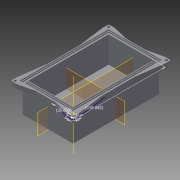
# Autodesk Inventor part: sensor3_2
Saved by Autodesk Inventor 2015 SP2 (Build 190223200, 223)
## iProperties
Created: 2016-02-03
Part Number: sensor3_2
Material: Generic
Document SubType Name: Modeling
Designer: mca20
Density: 1 g/cm^3
Appearance: Default
Author: mca20
Autodesk Inventor part; units mm, degrees
ref_plane "YZ Plane" through (0, 0, 0) normal (1, 0, 0) x (0, 1, 0)
ref_plane "XZ Plane" through (0, 0, 0) normal (0, 1, 0) x (-1, 0, 0)
ref_plane "XY Plane" through (0, 0, 0) normal (0, 0, 1) x (1, 0, 0)
sketch "Sketch1" plane through (0, 0, 0) normal (0, 1, 0) x (-1, 0, 0)
  line L0 (0, 0) -> (69.34, 0)
  line L1 (69.34, 0) -> (69.34, -118.083)
  line L2 (69.34, -118.083) -> (0, -118.083)
  line L3 (0, -118.083) -> (0, 0)
  dimension "d0" = 69.34
  dimension "d1" = 118.083
  constraints: 8 end point, 2 parallel, 1 horizontal, 1 perpendicular
  measures "d0" distance of L1.end L2.end
  measures "d1" distance of L0.end L1.end
extrude "Extrusion1" add sketch "Sketch1" along normal blind 1
sketch "Sketch2" plane through (0, 1, 0) normal (0, 1, 0) x (1, 0, 0)
  line L0 (0, 0) -> (0, 118.083) projected
  line L1 (-69.34, 0) -> (0, 0) projected
  line L2 (0, 0) -> (0, 118.083) projected
  line L3 (0, 118.083) -> (-69.34, 118.083) projected
  line L4 (-69.34, 118.083) -> (-69.34, 0) projected
  line L5 (-68.34, 1) -> (-1, 1)
  line L6 (-1, 1) -> (-1, 117.083)
  line L7 (-1, 117.083) -> (-68.34, 117.083)
  line L8 (-68.34, 117.083) -> (-68.34, 1)
  dimension "d4" = 1
  constraints: 8 end point, 3 other
  measures "d4" distance between parallel lines of L4 L8
extrude "Extrusion2" add sketch "Sketch2" along normal blind 35
sketch "Sketch3" plane through (0, 36, 0) normal (0, 1, 0) x (1, 0, 0)
  line L0 (-68.34, 1) -> (-68.34, 117.083) projected
  line L1 (-68.34, 117.083) -> (-1, 117.083) projected
  line L2 (-1, 117.083) -> (-1, 1) projected
  line L3 (-1, 1) -> (-68.34, 1) projected
  line L4 (-69.34, 0) -> (0, 0) projected
  line L5 (0, 0) -> (0, 118.083) projected
  line L6 (0, 118.083) -> (-69.34, 118.083) projected
  line L7 (-69.34, 118.083) -> (-69.34, 0) projected
  line L8 (-67.34, 116.083) -> (-67.34, 2)
  line L9 (-67.34, 2) -> (-2, 2)
  line L10 (-2, 2) -> (-2, 116.083)
  line L11 (-2, 116.083) -> (-67.34, 116.083)
  line L12 (-66.34, 3) -> (-66.34, 115.083)
  line L13 (-66.34, 115.083) -> (-3, 115.083)
  line L14 (-3, 115.083) -> (-3, 3)
  line L15 (-3, 3) -> (-66.34, 3)
  line L16 (-70.34, -1) -> (1, -1)
  line L17 (1, -1) -> (1, 119.083)
  line L18 (1, 119.083) -> (-70.34, 119.083)
  line L19 (-70.34, 119.083) -> (-70.34, -1)
  line L20 (-71.34, -2) -> (2, -2)
  line L21 (2, -2) -> (2, 120.083)
  line L22 (2, 120.083) -> (-71.34, 120.083)
  line L23 (-71.34, 120.083) -> (-71.34, -2)
  dimension "d7" = 1
  dimension "d8" = 1
  dimension "d9" = 1
  dimension "d10" = 1
  constraints: 32 end point, 12 other
  measures "d7" distance between parallel lines of L0 L8
  measures "d8" distance between parallel lines of L8 L12
  measures "d9" distance between parallel lines of L7 L19
  measures "d10" distance between parallel lines of L19 L23
extrude "Extrusion3" add sketch "Sketch3" along normal blind 1 contours L0 L1 L2 L3 | L7 L6 L5 L4 | L11 L10 L9 L8 | L19 L18 L17 L16 | L23 L22 L21 L20
sketch "Sketch4" plane through (0, 37, 0) normal (0, 1, 0) x (1, 0, 0)
  line L0 (-71.34, 120.083) -> (-71.34, -2) projected
  line L1 (-66.34, 3) -> (-66.34, 115.083) projected
  line L2 (-66.34, 115.083) -> (-3, 115.083) projected
  line L3 (-3, 115.083) -> (-3, 3) projected
  line L4 (-3, 3) -> (-66.34, 3) projected
  line L5 (-66.34, 3) -> (-66.34, 115.083) projected
  line L6 (-71.34, -2) -> (2, -2) projected
  line L7 (2, -2) -> (2, 120.083) projected
  line L8 (2, 120.083) -> (-71.34, 120.083) projected
  line L9 (-71.34, 120.083) -> (-71.34, -2) projected
  line L10 (-1, 1) -> (-68.34, 1) projected
  line L11 (-69.34, 0) -> (0, 0) projected
  line L12 (-69.34, 118.083) -> (-69.34, 0) projected
  line L13 (-68.34, 1) -> (-68.34, 117.083) projected
  line L14 (-1, 117.083) -> (-1, 1) projected
  line L15 (0, 0) -> (0, 118.083) projected
  line L16 (-68.34, 117.083) -> (-1, 117.083) projected
  line L17 (0, 118.083) -> (-69.34, 118.083) projected
  line L18 (-70.34, 119.083) -> (-70.34, -1)
  line L19 (-70.34, -1) -> (1, -1)
  line L20 (1, -1) -> (1, 119.083)
  line L21 (1, 119.083) -> (-70.34, 119.083)
  line L22 (-2, 116.083) -> (-67.34, 116.083)
  line L23 (-67.34, 116.083) -> (-67.34, 2)
  line L24 (-67.34, 2) -> (-2, 2)
  line L25 (-2, 2) -> (-2, 116.083)
  dimension "d13" = 1
  dimension "d14" = 1
  constraints: 16 end point, 6 other
  measures "d13" distance between parallel lines of L17 L21
  measures "d14" distance between parallel lines of L2 L22
extrude "Extrusion4" add sketch "Sketch4" along normal blind 1.5 contours L8 L7 L6 L0 | L25 L24 L23 L22
sketch "Sketch10" plane through (0, 37, 0) normal (0, 1, 0) x (1, 0, 0)
  line L0 (-71.34, -2) -> (2, -2) projected
  line L1 (-67.34, 2) -> (-2, 2) projected
  line L2 (-70.34, 119.083) -> (1, 119.083) projected
  line L3 (1, 119.083) -> (1, -1) projected
  line L4 (1, -1) -> (-70.34, -1) projected
  line L5 (-70.34, -1) -> (-70.34, 119.083) projected
  line L6 (-71.34, -2) -> (2, -2) projected
  line L7 (2, -2) -> (2, 120.083) projected
  line L8 (2, 120.083) -> (-71.34, 120.083) projected
  line L9 (-71.34, 120.083) -> (-71.34, -2) projected
  line L10 (-1, 1) -> (-68.34, 1) projected
  line L11 (-2, 116.083) -> (-2, 2) projected
  line L12 (-2, 2) -> (-67.34, 2) projected
  line L13 (-67.34, 2) -> (-67.34, 116.083) projected
  line L14 (-67.34, 116.083) -> (-2, 116.083) projected
  line L15 (1, 119.083) -> (-70.34, 119.083) projected
  line L16 (-70.34, 119.083) -> (-70.34, -1) projected
  line L17 (-70.34, -1) -> (1, -1) projected
  line L18 (1, -1) -> (1, 119.083) projected
  line L19 (-68.34, 1) -> (-68.34, 117.083) projected
  line L20 (-1, 117.083) -> (-1, 1) projected
  line L21 (1, 119.083) -> (1, -1) projected
  line L22 (0, 0) -> (0, 118.083) projected
  line L23 (-69.34, 0) -> (0, 0) projected
  line L24 (-69.34, 118.083) -> (-69.34, 0) projected
  line L25 (-2, 116.083) -> (-67.34, 116.083) projected
  line L26 (-68.34, 117.083) -> (-1, 117.083) projected
  line L27 (0, 118.083) -> (-69.34, 118.083) projected
  line L28 (-72.34, 121.083) -> (3, 121.083)
  line L29 (3, 121.083) -> (3, -3)
  line L30 (3, -3) -> (-72.34, -3)
  line L31 (-72.34, -3) -> (-72.34, 121.083)
  line L32 (-3, 115.083) -> (-3, 3) projected
  line L33 (-3, 3) -> (-66.34, 3) projected
  line L34 (-66.34, 3) -> (-66.34, 115.083) projected
  line L35 (-66.34, 115.083) -> (-3, 115.083) projected
  line L36 (-2, 116.083) -> (-67.34, 116.083) projected
  line L37 (-67.34, 116.083) -> (-67.34, 2) projected
  line L38 (-67.34, 2) -> (-2, 2) projected
  line L39 (-2, 2) -> (-2, 116.083) projected
  line L40 (-65.34, 114.083) -> (-65.34, 4)
  line L41 (-65.34, 4) -> (-4, 4)
  line L42 (-4, 4) -> (-4, 114.083)
  line L43 (-4, 114.083) -> (-65.34, 114.083)
  dimension "d50" = 1
  dimension "d51" = 1
  dimension "d69" = 61.34
  dimension "d70" = 110.083
  constraints: 16 end point, 6 other
  measures "d50" distance between parallel lines of L8 L28
  measures "d51" distance between parallel lines of L34 L40
  measures "d69" distance between parallel lines of L42 L40
  measures "d70" distance between parallel lines of L41 L43
extrude "Extrusion6" add sketch "Sketch10" along normal blind 3 and the other way blind 1 contours L28 L29 L30 L31 | L32 L33 L34 L35
sketch "Sketch5" plane through (0, 36, 0) normal (0, -1, 0) x (1, 0, 0)
  line L0 (0, 0) -> (8, 0)
  line L1 (8, 0) -> (8, 8)
  line L2 (8, 8) -> (0, 8)
  line L3 (0, 8) -> (0, 0)
  line L4 (8, 8) -> (2, 8)
  line L5 (2, 8) -> (2, 2)
  line L6 (2, 2) -> (8, 2)
  line L7 (8, 2) -> (8, 8)
  line L8 (0, 0) -> (0, -118.083) projected
  line L9 (0, -59.0415) -> (8, 0)
  line L10 (-69.34, 0) -> (0, 0) projected
  line L11 (-34.67, 0) -> (0, 8)
  circle A0 centre (5, 5) radius 1.5
  line L12 (7, 3) -> (3, 3)
  line L13 (3, 3) -> (3, 7)
  line L14 (3, 7) -> (7, 7)
  line L15 (7, 7) -> (7, 3)
  line L16 (-71.34, 2) -> (2, 2) projected
  line L17 (-26.0025, 2) -> (-26.0025, 0)
  line L18 (-26.0025, 2) -> (-16.75, 2) construction
  dimension "d17" = 8
  dimension "d18" = 8
  dimension "d21" = 6
  dimension "d29" = 118.083
  dimension "d31" = 3
  dimension "d32" = 1
  dimension "d47" = 26.0025
  constraints: 32 end point, 6 parallel, 4 perpendicular, 3 horizontal, 3 point on line, 2 midpoint, 1 centre point, 1 coincident, 3 other
  measures "d17" distance of L2.end L1.end
  measures "d18" distance of L1.end L0.end
  measures "d21" distance between parallel lines of L2 L6
  measures "d29" distance of L0.start L8.end
  measures "d31" diameter of A0
  measures "d32" distance between parallel lines of L6 L12
  measures "d47" distance between parallel lines of L3 L17
extrude "Extrusion5" add sketch "Sketch5" along normal blind 2 contours L3 L16 L6 L1 L0 | L10 L17 L16 L3 | L0 L9 L8 | L16 L11 L3 | L3 L2 L5 L16 | L10 L11 L17 | L6 L5 L2 L1 | A0 | L12 L13 L14 L15
sketch "Sketch6" plane through (0, 36, 0) normal (0, 1, 0) x (1, 0, 0)
  line L0 (8, -8) -> (0, -8) projected
  line L1 (8, -8) -> (0, -8) projected
  line L2 (8, 0) -> (8, -8) projected
  line L3 (8, -8) -> (2, -8)
  line L4 (2, -8) -> (2, -2)
  line L5 (2, -2) -> (8, -2)
  line L6 (8, -2) -> (8, -8)
  line L7 (0, -8) -> (-21.6687, -3) projected
  line L8 (3, 36.9009) -> (8, 0) projected
  line L9 (3, 36.9009) -> (3, -3) projected
  line L10 (3, -3) -> (-21.6687, -3) projected
  point P0 (0, 0)
  point P1 (5, -5)
  dimension "d33" = 3
  dimension "d34" = 6
  dimension "d35" = 3
  dimension "d36" = 3
  constraints: 8 end point, 2 parallel, 1 horizontal, 1 perpendicular
  measures "d33" distance from line of L5 point (5, -5)
  measures "d34" distance between parallel lines of L5 L0
  measures "d35" distance from line of L2 point (5, -5)
  measures "d36" distance from line of L0 point (5, -5)
hole "Hole1" at (5, 36, 5) direction (0, -1, 0) diameter 3 end through all
fillet "Fillet1" radius 2 1 edges at (8, 35, 8)
sketch "Sketch11" plane through (0, 36, 0) normal (0, 1, 0) x (1, 0, 0)
  line L0 (8, -8) -> (2, -8)
  line L1 (2, -8) -> (2, -2)
  line L2 (2, -2) -> (8, -2)
  line L3 (8, -2) -> (8, -8)
  line L4 (0, 0) -> (8, 0)
  line L5 (8, 0) -> (8, -8)
  line L6 (8, -8) -> (0, -8)
  line L7 (0, -8) -> (0, 0)
  line L8 (-21.6687, -3) -> (0, -8)
  line L9 (0, -8) -> (-21.6687, -3) projected
  line L10 (-21.6687, -3) -> (0, -3)
  line L11 (3, -3) -> (-21.6687, -3) projected
  line L12 (3, -2) -> (3, 36.9009)
  line L13 (3, 36.9009) -> (8, 0)
  line L14 (3, -3) -> (3, -2)
  line L15 (3, 36.9009) -> (3, -3) projected
  dimension "d56" = 6
  dimension "d57" = 6
  constraints: 26 end point, 4 parallel, 3 point on line, 2 collinear, 2 horizontal, 2 perpendicular, 1 vertical
  measures "d56" distance of L1.end L2.end
  measures "d57" distance of L0.end L1.end
extrude "Extrusion7" add sketch "Sketch11" along normal blind 4 contours L0 L1 L11 L14 L2 L3 | L6 L7 L11 L1 | L2 L12 L4 L5 | L8 L10 L7 | L4 L12 L13
fillet "Fillet2" radius 2 1 edges at (8, 38, 8)
sketch "Sketch12" plane through (0, 40, 0) normal (0, 1, 0) x (1, 0, 0)
  circle A0 centre (5, -5) radius 1.5 projected
  point P0 (0, 0)
  dimension "d61" = 3
  measures "d61" diameter of A0
hole "Hole2" at (5, 40, 5) direction (0, -1, 0) diameter 3 end through all
ref_plane "Work Plane1" through (0, 0, 0) normal (0.7071068, 0, -0.7071068) x (0, 1, 0)
ref_plane "Work Plane5" through (-69.34, 0, -59.0415) normal (0, 0, 1) x (1, 0, 0)
ref_plane "Work Plane6" through (-34.67, 0, 0) normal (1, 0, 0) x (0, 0, -1)
mirror "Mirror6" about plane through (-69.34, 0, -59.0415) normal (0, 0, 1) of "Extrusion5", "Hole1", "Fillet1", "Extrusion7", "Fillet2", "Hole2"
mirror "Mirror7" about plane through (-34.67, 0, 0) normal (1, 0, 0) of "Extrusion5", "Hole1", "Fillet1", "Extrusion7", "Fillet2", "Hole2", "Mirror6"
body "Solid1"
